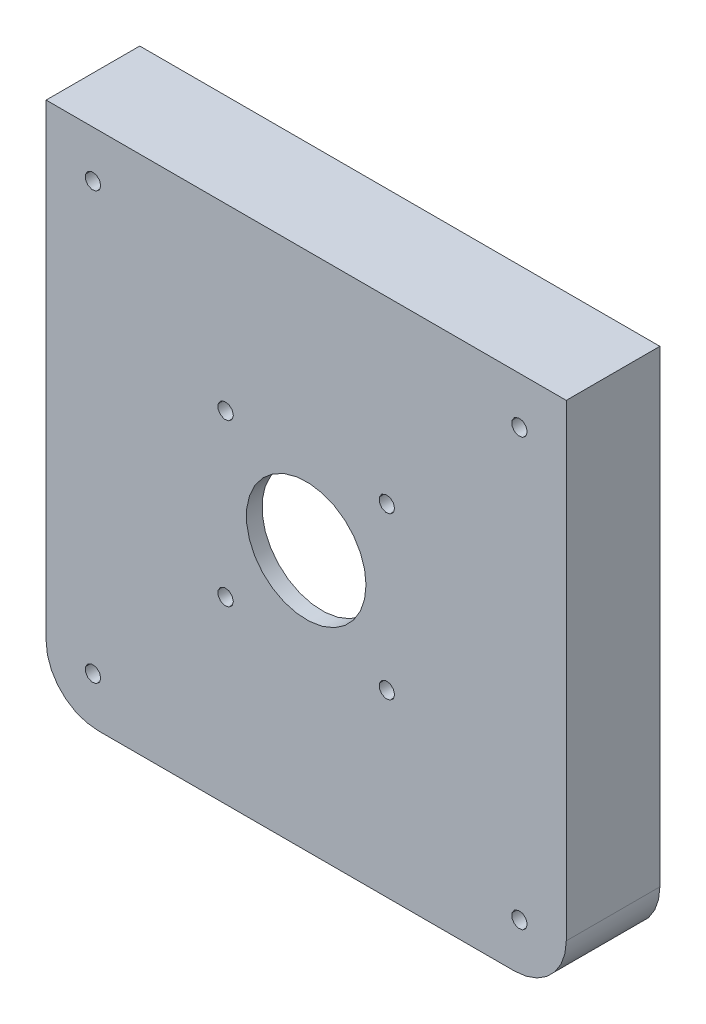
# Autodesk Inventor part: Cup_Dispenser_Stepper_Montage
Saved by Autodesk Inventor 2016 (Build 200138000, 138)
## iProperties
Created: 2015-07-09
Part Number: Cup_Dispenser_Stepper_Montage
Material: Generic
Document SubType Name: Modeling
Designer: marku
Density: 1 g/cm^3
Appearance: Default
Author: marku
Autodesk Inventor part; units mm, degrees
ref_plane "YZ Plane" through (0, 0, 0) normal (1, 0, 0) x (0, 1, 0)
ref_plane "XZ Plane" through (0, 0, 0) normal (0, 1, 0) x (-1, 0, 0)
ref_plane "XY Plane" through (0, 0, 0) normal (0, 0, 1) x (1, 0, 0)
sketch "Sketch1" plane through (0, 0, 0) normal (0, 0, 1) x (1, 0, 0)
  circle A0 centre (-41, -93.7922) radius 1.5 projected
  circle A1 centre (41, -93.7922) radius 1.5 projected
  circle A2 centre (-41, 88.2078) radius 1.5 projected
  circle A3 centre (41, 6.2078) radius 1.5 projected
  circle A4 centre (41, 88.2078) radius 1.5 projected
  circle A5 centre (-41, 6.2078) radius 1.5 projected
  circle A6 centre (41, -11.7922) radius 1.5 projected
  circle A7 centre (-41, -11.7922) radius 1.5 projected
  circle A8 centre (0, -52.7922) radius 47 projected
  circle A9 centre (0, 47.2078) radius 47 projected
  line L0 (-50, 97.2078) -> (-50, -92.7922) projected
  arc A10 (-50, -92.7922) -> (-40, -102.7922) centre (-40, -92.7922) ccw projected
  line L1 (-40, -102.7922) -> (40, -102.7922) projected
  arc A11 (40, -102.7922) -> (50, -92.7922) centre (40, -92.7922) ccw projected
  line L2 (50, -92.7922) -> (50, 97.2078) projected
  line L3 (50, 97.2078) -> (-50, 97.2078) projected
  line L4 (-50, -2.7922) -> (50, -2.7922) projected
  point P0 (0, 0)
extrude "Extrusion1" add sketch "Sketch1" along normal blind 15 contours L4 L2 A11 L1 A10 L0
sketch "Sketch2" plane through (0, 0, 15) normal (0, 0, 1) x (1, 0, 0)
  circle A0 centre (0, -52.7922) radius 47 projected
  circle A1 centre (-41, -11.7922) radius 1.5 projected
  circle A2 centre (41, -11.7922) radius 1.5 projected
  circle A3 centre (41, -93.7922) radius 1.5 projected
  circle A4 centre (-41, -93.7922) radius 1.5 projected
  arc A5 (-50, -92.7922) -> (-40, -102.7922) centre (-40, -92.7922) ccw projected
  line L0 (-40, -102.7922) -> (40, -102.7922) projected
  arc A6 (40, -102.7922) -> (50, -92.7922) centre (40, -92.7922) ccw projected
  line L1 (50, -92.7922) -> (50, -2.7922) projected
  line L2 (50, -2.7922) -> (-50, -2.7922) projected
  line L3 (-50, -2.7922) -> (-50, -92.7922) projected
  point P0 (0, 0)
extrude "Extrusion2" add sketch "Sketch2" along normal blind 3 contours A0 | L3 L2 L1 A6 L0 A5
sketch "Sketch3" plane through (0, 0, 18) normal (0, 0, 1) x (1, 0, 0)
  circle A0 centre (0, -52.7922) radius 47 projected
  circle A1 centre (0, -52.7922) radius 11.5
  point P0 (0, 0)
  dimension "d4" = 23
  constraints: 1 centre point, 1 coincident
  measures "d4" diameter of A1
extrude "Extrusion3" cut sketch "Sketch3" against normal up to next contours A1
sketch "Sketch4" plane through (0, 0, 18) normal (0, 0, 1) x (1, 0, 0)
  circle A0 centre (0, -52.7922) radius 11.5 construction
  line L0 (-15.5, -37.2922) -> (15.5, -37.2922) construction
  line L1 (15.5, -37.2922) -> (15.5, -68.2922) construction
  line L2 (15.5, -68.2922) -> (-15.5, -68.2922) construction
  line L3 (-15.5, -68.2922) -> (-15.5, -37.2922) construction
  line L4 (-15.5, -37.2922) -> (15.5, -68.2922) construction
  line L5 (15.5, -37.2922) -> (-15.5, -68.2922) construction
  point P0 (0, 0)
  dimension "d7" = 31
  dimension "d8" = 31
  constraints: 12 end point, 4 coincident, 2 midpoint, 2 parallel, 1 horizontal, 1 perpendicular
  measures "d7" distance of L1.end L2.end
  measures "d8" distance of L0.end L1.end
hole "Hole1" at (15.5, -68.2922, 18) at (-15.5, -68.2922, 18) at (-15.5, -37.2922, 18) at (15.5, -37.2922, 18) direction (0, 0, -1) diameter 3 depth 8 tip angle 118
equation "\"d0\" = 5 * thickness"
equation "\"d2\" = thickness"
equation "\"d5\" = thickness"
equation "\"thickness\" = 3"
body "Solid1"
